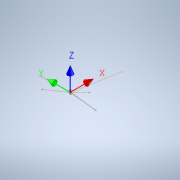
# Autodesk Inventor part: Coupler
Saved by Autodesk Inventor 2020.1 (Build 241239000, 239)
## iProperties
Created: 2019-10-25
Part Number: Coupler
Material: Generic
Document SubType Name: Modeling
Designer: sshel
Density: 1 g/cm^3
Appearance: Default
Mass: 190025 g
Surface Area: 74701 cm^2
Volume: 190025 cm^3
Author: sshel
Autodesk Inventor part; units mm, degrees
ref_plane "YZ Plane" through (0, 0, 0) normal (1, 0, 0) x (0, 1, 0)
ref_plane "XZ Plane" through (0, 0, 0) normal (0, 1, 0) x (-1, 0, 0)
ref_plane "XY Plane" through (0, 0, 0) normal (0, 0, 1) x (1, 0, 0)
ref_plane "Dyad1 plane" through (-3690.83, 3605.1, 722.841) normal (-0.708447, 0.6919913, 0.1387478) x (-0.6987498, -0.7153662, 0)
sketch "Sketch3" plane through (-3690.83, 3605.1, 722.841) normal (-0.708447, 0.6919913, 0.1387478) x (-0.6987498, -0.7153662, 0)
  circle A0 centre (0, 0) radius 100
  point P0 (0, 0)
  dimension "d16" = 100
  constraints: 1 centre point, 1 coincident
  measures "d16" radius of A0
sketch3d "import_point_3Dsketch"
  line L0 (-3690.83, 3605.1, 722.841) -> (0, 0, 0)
sweep "Dyad1 rod" add profiles "Sketch3" path "import_point_3Dsketch"
sketch "Sketch2" plane through (-3690.83, 3605.1, 722.841) normal (-0.708447, 0.6919913, 0.1387478) x (-0.6987498, -0.7153662, 0)
  circle A0 centre (0, 0) radius 200
  line L0 (200, 0) -> (-200, 0)
  point P0 (0, 0)
  dimension "d17" = 200
  constraints: 2 end point, 2 point on circle, 1 centre point, 1 coincident, 1 horizontal, 1 midpoint
  measures "d17" radius of A0
revolve "Dyad1 joint" add sketch "Sketch2" angle 360 about axis through (-3830.58, 3462.0268, 722.841) along (0.6987498, 0.7153662, 0) separate body picked at (-37.038, -55.4313) contours A0 L0
ref_plane "Dyad2 plane" through (4881.45, -1551.69, -5595.43) normal (0.6434941, -0.2045506, -0.737614) x (0.302938, 0.9530103, 0)
sketch "Sketch4" plane through (4881.45, -1551.69, -5595.43) normal (0.6434941, -0.2045506, -0.737614) x (0.302938, 0.9530103, 0)
  circle A0 centre (0, 0) radius 100
  point P0 (0, 0)
  dimension "d14" = 100
  constraints: 1 centre point, 1 coincident
  measures "d14" radius of A0
sketch3d "import_point_3Dsketch for Dyad2 rod"
  line L0 (4881.45, -1551.69, -5595.43) -> (0, 0, 0)
sweep "Dyad2 rod" add profiles "Sketch4" path "import_point_3Dsketch for Dyad2 rod" separate body
sketch "Sketch5" plane through (4881.45, -1551.69, -5595.43) normal (0.6434941, -0.2045506, -0.737614) x (0.302938, 0.9530103, 0)
  circle A0 centre (0, 0) radius 200
  line L0 (200, 0) -> (-200, 0)
  point P0 (0, 0)
  dimension "d11" = 200
  constraints: 2 end point, 2 point on circle, 1 centre point, 1 coincident, 1 horizontal, 1 midpoint
  measures "d11" radius of A0
revolve "Dyad2 joint" add sketch "Sketch5" angle 360 about axis through (4942.0376, -1361.0879, -5595.43) along (-0.302938, -0.9530103, 0) picked at (-37.038, -55.4313) bodies 2 contours A0 L0
ref_plane "Dyad3 plane" through (-7397.93, 538.118, 7168.14) normal (-0.7171946, 0.052168, 0.6949175) x (-0.0725473, -0.997365, 0)
sketch "Sketch6" plane through (-7397.93, 538.118, 7168.14) normal (-0.7171946, 0.052168, 0.6949175) x (-0.0725473, -0.997365, 0)
  circle A0 centre (0, 0) radius 100
  point P0 (0, 0)
  dimension "d18" = 100
  constraints: 1 centre point, 1 coincident
  measures "d18" radius of A0
sketch3d "import_point_3Dsketch for Dyad3 rod"
  line L0 (-7397.93, 538.118, 7168.14) -> (0, 0, 0)
sweep "Dyad3 rod" add profiles "Sketch6" path "import_point_3Dsketch for Dyad3 rod" separate body
sketch "Sketch7" plane through (-7397.93, 538.118, 7168.14) normal (-0.7171946, 0.052168, 0.6949175) x (-0.0725473, -0.997365, 0)
  circle A0 centre (0, 0) radius 200
  line L0 (200, 0) -> (-200, 0)
  point P0 (0, 0)
  dimension "d21" = 200
  constraints: 2 end point, 2 point on circle, 1 centre point, 1 coincident, 1 horizontal, 1 midpoint
  measures "d21" radius of A0
revolve "Dyad3 joint" add sketch "Sketch7" angle 360 about axis through (-7412.4395, 338.645, 7168.14) along (0.0725473, 0.997365, 0) picked at (-37.038, -55.4313) bodies 2 contours A0 L0
ref_plane "Dyad4 plane" through (689.914, -4215.56, 1695.37) normal (0.150119, -0.9172673, 0.368897) x (0.986871, 0.1615102, 0)
sketch "Sketch8" plane through (689.914, -4215.56, 1695.37) normal (0.150119, -0.9172673, 0.368897) x (0.986871, 0.1615102, 0)
  circle A0 centre (0, 0) radius 100
  point P0 (0, 0)
  dimension "d23" = 100
  constraints: 1 centre point, 1 coincident
  measures "d23" radius of A0
sketch3d "import_point_3Dsketch for Dyad4 rod"
  line L0 (689.914, -4215.56, 1695.37) -> (0, 0, 0)
sweep "Dyad4 rod" add profiles "Sketch8" path "import_point_3Dsketch for Dyad4 rod" separate body
sketch "Sketch9" plane through (689.914, -4215.56, 1695.37) normal (0.150119, -0.9172673, 0.368897) x (0.986871, 0.1615102, 0)
  circle A0 centre (0, 0) radius 200
  line L0 (200, 0) -> (-200, 0)
  point P0 (0, 0)
  dimension "d26" = 200
  constraints: 2 end point, 2 point on circle, 1 centre point, 1 coincident, 1 horizontal, 1 midpoint
  measures "d26" radius of A0
revolve "Dyad4 joint" add sketch "Sketch9" angle 360 about axis through (887.2882, -4183.258, 1695.37) along (-0.986871, -0.1615102, 0) picked at (-37.038, -55.4313) bodies 2 contours A0 L0
ref_plane "Dyad5 plane" through (-2857.82, -16145.8, 14116.3) normal (-0.1320853, -0.7462411, 0.6524398) x (0.9846941, -0.1742917, 0)
sketch "Sketch10" plane through (-2857.82, -16145.8, 14116.3) normal (-0.1320853, -0.7462411, 0.6524398) x (0.9846941, -0.1742917, 0)
  circle A0 centre (0, 0) radius 100
  point P0 (0, 0)
  dimension "d28" = 100
  constraints: 1 centre point, 1 coincident
  measures "d28" radius of A0
sketch3d "import_point_3Dsketch for Dyad5 rod"
  line L0 (-2857.82, -16145.8, 14116.3) -> (0, 0, 0)
sweep "Dyad5 rod" add profiles "Sketch10" path "import_point_3Dsketch for Dyad5 rod" separate body
sketch "Sketch11" plane through (-2857.82, -16145.8, 14116.3) normal (-0.1320853, -0.7462411, 0.6524398) x (0.9846941, -0.1742917, 0)
  circle A0 centre (0, 0) radius 200
  line L0 (200, 0) -> (-200, 0)
  point P0 (0, 0)
  dimension "d31" = 200
  constraints: 2 end point, 2 point on circle, 1 centre point, 1 coincident, 1 horizontal, 1 midpoint
  measures "d31" radius of A0
revolve "Dyad5 joint" add sketch "Sketch11" angle 360 about axis through (-2660.8812, -16180.6583, 14116.3) along (-0.9846941, 0.1742917, 0) picked at (-37.038, -55.4313) bodies 2 contours A0 L0
combine bodies "Combine1" operation type add bodies to combine 1 2 3 4 5 6
sketch "Sketch12" plane through (0, 0, 0) normal (0, 0, 1) x (1, 0, 0)
  circle A0 centre (0, 0) radius 200
  line L0 (-200, 0) -> (200, 0)
  dimension "d33" = 400
  constraints: 2 end point, 2 point on circle, 1 centre point, 1 coincident, 1 horizontal, 1 midpoint
  measures "d33" diameter of A0
revolve "Revolution7" add sketch "Sketch12" angle 360 about axis through (-200, 0, 0) along (1, 0, 0) picked at (-37.038, -55.4313) bodies 1 contours A0 L0
equation "\"d16\" = rod_radius"
equation "\"d17\" = S_radius"
equation "\"d14\" = rod_radius"
equation "\"d11\" = S_radius"
equation "\"d18\" = rod_radius"
equation "\"d21\" = S_radius"
equation "\"d23\" = rod_radius"
equation "\"d26\" = S_radius"
equation "\"d28\" = rod_radius"
equation "\"d31\" = S_radius"
equation "\"d33\" = 2 * S_radius"
equation "\"rod_radius\" = 100"
equation "\"S_radius\" = 2 * rod_radius"
body "Solid3"
